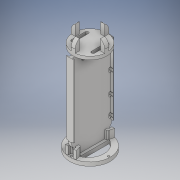
# Autodesk Inventor part: Platform_v1
Saved by Autodesk Inventor 2017 (Build 210142000, 142)
## iProperties
Created: 2018-06-09
Part Number: Platform_v1
Material: Generic
Document SubType Name: Modeling
Designer: Arthur
Density: 1 g/cm^3
Appearance: Default
Author: Arthur
Autodesk Inventor part; units mm, degrees
ref_plane "YZ Plane" through (0, 0, 0) normal (1, 0, 0) x (0, 1, 0)
ref_plane "XZ Plane" through (0, 0, 0) normal (0, 1, 0) x (-1, 0, 0)
ref_plane "XY Plane" through (0, 0, 0) normal (0, 0, 1) x (1, 0, 0)
sketch "Sketch3" plane through (0, 0, 0) normal (0, 1, 0) x (-1, 0, 0)
  circle A0 centre (0, 0) radius 37.75
  circle A1 centre (-34.675, 0) radius 1.9
  circle A2 centre (0, 34.675) radius 1.9
  circle A3 centre (34.675, 0) radius 1.9
  circle A4 centre (0, -34.675) radius 1.9
  line L0 (8, -27.7356) -> (8, 27.5985)
  arc A5 (8, -27.7356) -> (8, 27.5985) centre (-3.5989, -0.0685) ccw
  line L1 (-8, -27.7356) -> (-8, 27.5985)
  arc A6 (-8, 27.5985) -> (-8, -27.7356) centre (3.5989, -0.0685) ccw
  dimension "d3" = 3.8
  dimension "d7" = 3.8
  dimension "d9" = 3.8
  dimension "d33" = 30
  constraints: 7 centre point, 4 end point, 4 point on circle, 2 vertical
  measures "d3" diameter of A1
  measures "d7" diameter of A3
  measures "d9" diameter of A4
  measures "d33" radius of A6
extrude "Extrusion1" add sketch "Sketch3" along normal blind 7
sketch "Sketch4" plane through (0, 7, 0) normal (0, 1, 0) x (1, 0, 0)
  line L0 (-3, -30) -> (3, -30)
  line L1 (3, -24.5985) -> (3, 24.7356)
  line L2 (3, 30) -> (-3, 30)
  line L3 (-3, 24.7356) -> (-3, -24.2326)
  line L4 (-3, -30) -> (3, 30) construction
  line L5 (3, -30) -> (-3, 30) construction
  line L6 (-3, 30) -> (-5, 30)
  line L7 (-5, 30) -> (-5, 36)
  line L8 (-5, 36) -> (-10, 36)
  line L9 (-8, 27.7356) -> (-8, -27.5985) projected
  line L10 (-10, 36) -> (-8, 27.7356)
  line L11 (-3, -30) -> (-5, -30)
  line L12 (-5, -30) -> (-5, -36)
  line L13 (-5, -36) -> (-10, -36)
  line L14 (-10, -36) -> (-8, -27.2326)
  line L15 (-8, -27.2326) -> (-8, -24.2326)
  line L16 (-8, -24.2326) -> (-3, -24.2326)
  line L17 (-8, 27.7356) -> (-8, 24.7356)
  line L18 (-8, 24.7356) -> (-3, 24.7356)
  line L19 (3, -30) -> (5, -30)
  line L20 (5, -30) -> (5, -36)
  line L21 (5, -36) -> (10, -36)
  line L22 (10, -36) -> (8, -27.5985)
  line L23 (8, -27.5985) -> (8, -24.5985)
  line L24 (8, -27.5985) -> (8, 27.7356) projected
  line L25 (8, -24.5985) -> (5, -24.5985)
  line L26 (3, 30) -> (5, 30)
  line L27 (5, 30) -> (5, 36)
  line L28 (5, 36) -> (10, 36)
  line L29 (10, 36) -> (8, 27.7356)
  line L30 (8, 24.7356) -> (3, 24.7356)
  line L31 (5, -24.5985) -> (3, -24.5985)
  point P0 (0, 0)
  dimension "d36" = 6
  dimension "d37" = 60
  dimension "d38" = 2
  dimension "d39" = 6
  dimension "d40" = 5
  dimension "d41" = 6
  dimension "d42" = 5
  dimension "d43" = 3
  dimension "d44" = 3
  dimension "d45" = 2
  dimension "d46" = 5
  dimension "d47" = 3
  dimension "d48" = 2
  constraints: 60 end point, 13 perpendicular, 6 horizontal, 5 point on line, 2 midpoint, 2 parallel
  measures "d36" distance of L2.end L2.start
  measures "d37" distance of L2.start L0.end
  measures "d38" distance of L2.end L6.end
  measures "d39" distance of L6.end L7.end
  measures "d40" distance of L7.end L8.end
  measures "d41" distance of L11.end L12.end
  measures "d42" distance of L12.end L13.end
  measures "d43" distance of L14.end L15.end
  measures "d44" distance of L9.start L17.end
  measures "d45" distance of L0.end L19.end
  measures "d46" distance of L20.end L21.end
  measures "d47" distance of L22.end L23.end
  measures "d48" distance of L2.start L26.end
extrude "Extrusion2" add sketch "Sketch4" along normal blind 15 contours L11 L12 L13 L14 L9 L16 L3 L18 L10 L8 L7 L6 L2 L26 L27 L28 L29 L24 L30 L1 L31 L25 L23 L22 L21 L20 L19 L0
fillet "Fillet1" radius 2 1 edges at (-5, 14.5, 30)
fillet "Fillet2" radius 2 1 edges at (5, 14.5, 30)
fillet "Fillet3" radius 2 1 edges at (-5, 14.5, -30)
fillet "Fillet4" radius 2 1 edges at (5, 14.5, -30)
fillet "Fillet5" radius 2 1 edges at (-8, 14.5, -24.7356)
fillet "Fillet6" radius 2 1 edges at (8, 14.5, -24.7356)
fillet "Fillet7" radius 2 1 edges at (8, 14.5, 24.5985)
fillet "Fillet8" radius 2 1 edges at (-8, 14.5, 24.2326)
sketch "Sketch5" plane through (0, 22, 0) normal (0, 1, 0) x (1, 0, 0)
  circle A0 centre (0, 0) radius 37.75 projected
  line L0 (3, -37.6306) -> (3, 37.6306)
  line L1 (-3, 37.6306) -> (-3, -37.6306)
  arc A1 (-3, -37.6306) -> (3, -37.6306) centre (0, 0) ccw
  arc A2 (3, 37.6306) -> (-3, 37.6306) centre (0, 0) ccw
  constraints: 4 end point, 4 point on circle, 2 centre point, 1 coincident, 1 parallel, 2 other
extrude "Extrusion3" add sketch "Sketch5" along normal blind 146 contours L0 A0 L1
fillet "Fillet9" radius 7 1 edges at (0, 22, 30)
fillet "Fillet10" radius 7 1 edges at (0, 22, -30)
fillet "Fillet11" radius 15 1 edges at (0, 22, 37.75)
fillet "Fillet12" radius 15 1 edges at (0, 22, -37.75)
sketch "Sketch8" plane through (0, 168, 0) normal (0, 1, 0) x (1, 0, 0)
  circle A0 centre (0, 0) radius 31.6345
  constraints: 1 centre point, 1 coincident
extrude "Extrusion5" add sketch "Sketch8" along normal blind 6
sketch "Sketch10" plane through (0, 168, 0) normal (0, -1, 0) x (1, 0, 0)
  line L0 (-7, 37.0953) -> (-7, 36.1306)
  line L1 (-7, 36.1306) -> (-3, 36.1306)
  line L2 (-3, 36.1306) -> (-3, 37.6306)
  line L3 (7, 37.0953) -> (7, 36.1306)
  line L4 (7, 36.1306) -> (3, 36.1306)
  line L5 (3, 36.1306) -> (3, 37.6306)
  line L6 (7, -37.0953) -> (7, -36.1306)
  line L7 (7, -36.1306) -> (3, -36.1306)
  line L8 (3, -36.1306) -> (3, -37.6306)
  line L9 (-7, -37.0953) -> (-7, -36.1306)
  line L10 (-7, -36.1306) -> (-3, -36.1306)
  line L11 (-3, -36.1306) -> (-3, -37.6306)
  arc A0 (7, 37.0953) -> (3, 37.6306) centre (0, 0) ccw
  arc A1 (-3, 37.6306) -> (-7, 37.0953) centre (0, 0) ccw
  arc A2 (-7, -37.0953) -> (-3, -37.6306) centre (0, 0) ccw
  arc A3 (3, -37.6306) -> (7, -37.0953) centre (0, 0) ccw
  constraints: 24 end point, 8 point on circle, 4 centre point, 4 parallel, 1 coincident
extrude "Extrusion7" add sketch "Sketch10" along normal blind 135
sketch "Sketch11" plane through (-3, 7, -24.7356) normal (-1, 0, 0) x (0, 0, 1)
  line L0 (60.8662, 26) -> (61.8309, 26) projected
  line L1 (58.8662, 31) -> (58.8662, 36) construction
  line L2 (60.8662, 31) -> (60.8662, 36)
  line L3 (56.8662, 36) -> (56.8662, 31)
  arc A0 (56.8662, 31) -> (60.8662, 31) centre (58.8662, 31) ccw
  arc A1 (60.8662, 36) -> (56.8662, 36) centre (58.8662, 36) ccw
  line L4 (-9.5219, 31) -> (-9.5219, 36) construction
  line L5 (-7.5219, 31) -> (-7.5219, 36)
  line L6 (-11.5219, 36) -> (-11.5219, 31)
  arc A2 (-11.5219, 31) -> (-7.5219, 31) centre (-9.5219, 31) ccw
  arc A3 (-7.5219, 36) -> (-11.5219, 36) centre (-9.5219, 36) ccw
  line L7 (58.8662, 65.1959) -> (58.8662, 70.1959) construction
  line L8 (60.8662, 65.1959) -> (60.8662, 70.1959)
  line L9 (56.8662, 70.1959) -> (56.8662, 65.1959)
  arc A4 (56.8662, 65.1959) -> (60.8662, 65.1959) centre (58.8662, 65.1959) ccw
  arc A5 (60.8662, 70.1959) -> (56.8662, 70.1959) centre (58.8662, 70.1959) ccw
  line L10 (-9.5219, 65.1959) -> (-9.5219, 70.1959) construction
  line L11 (-7.5219, 65.1959) -> (-7.5219, 70.1959)
  line L12 (-11.5219, 70.1959) -> (-11.5219, 65.1959)
  arc A6 (-11.5219, 65.1959) -> (-7.5219, 65.1959) centre (-9.5219, 65.1959) ccw
  arc A7 (-7.5219, 70.1959) -> (-11.5219, 70.1959) centre (-9.5219, 70.1959) ccw
  line L13 (58.8662, 104.699) -> (58.8662, 109.699) construction
  line L14 (60.8662, 104.699) -> (60.8662, 109.699)
  line L15 (56.8662, 109.699) -> (56.8662, 104.699)
  arc A8 (56.8662, 104.699) -> (60.8662, 104.699) centre (58.8662, 104.699) ccw
  arc A9 (60.8662, 109.699) -> (56.8662, 109.699) centre (58.8662, 109.699) ccw
  line L16 (-9.5219, 104.699) -> (-9.5219, 109.699) construction
  line L17 (-7.5219, 104.699) -> (-7.5219, 109.699)
  line L18 (-11.5219, 109.699) -> (-11.5219, 104.699)
  arc A10 (-11.5219, 104.699) -> (-7.5219, 104.699) centre (-9.5219, 104.699) ccw
  arc A11 (-7.5219, 109.699) -> (-11.5219, 109.699) centre (-9.5219, 109.699) ccw
  line L19 (58.8662, 144.202) -> (58.8662, 149.202) construction
  line L20 (60.8662, 144.202) -> (60.8662, 149.202)
  line L21 (56.8662, 149.202) -> (56.8662, 144.202)
  arc A12 (56.8662, 144.202) -> (60.8662, 144.202) centre (58.8662, 144.202) ccw
  arc A13 (60.8662, 149.202) -> (56.8662, 149.202) centre (58.8662, 149.202) ccw
  line L22 (-9.5219, 144.202) -> (-9.5219, 149.202) construction
  line L23 (-7.5219, 144.202) -> (-7.5219, 149.202)
  line L24 (-11.5219, 149.202) -> (-11.5219, 144.202)
  arc A14 (-11.5219, 144.202) -> (-7.5219, 144.202) centre (-9.5219, 144.202) ccw
  arc A15 (-7.5219, 149.202) -> (-11.5219, 149.202) centre (-9.5219, 149.202) ccw
  point P0 (24.7356, -7)
  point P1 (58.8662, 33.5)
  point P2 (-9.5219, 33.5)
  point P3 (58.8662, 67.6959)
  point P4 (-9.5219, 67.6959)
  point P5 (58.8662, 107.199)
  point P6 (-9.5219, 107.199)
  point P7 (58.8662, 146.702)
  point P8 (-9.5219, 146.702)
  dimension "d90" = 5
  dimension "d91" = 4
  dimension "d94" = 4
  dimension "d95" = 5
  dimension "d96" = 4
  dimension "d97" = 4
  dimension "d98" = 5
  dimension "d99" = 4
  dimension "d100" = 4
  dimension "d101" = 5
  dimension "d102" = 4
  dimension "d103" = 4
  constraints: 64 end point, 32 point on circle, 32 tangent, 16 centre point, 8 midpoint, 8 parallel, 8 vertical
  measures "d90" distance of L1.start L1.end
  measures "d91" diameter of A1
  measures "d94" diameter of A3
  measures "d95" distance of L7.start L7.end
  measures "d96" diameter of A5
  measures "d97" diameter of A7
  measures "d98" distance of L13.start L13.end
  measures "d99" diameter of A9
  measures "d100" diameter of A11
  measures "d101" distance of L19.start L19.end
  measures "d102" diameter of A13
  measures "d103" diameter of A15
extrude "Extrusion8" cut sketch "Sketch11" against normal through all
sketch "Sketch13" plane through (0, 174, 0) normal (0, 1, 0) x (1, 0, 0)
  circle A0 centre (0, 0) radius 31.6345 projected
  line L0 (-23.6093, -3.9201) -> (-31.3907, -3.9201)
  line L1 (-31.3907, 3.9201) -> (-23.6093, 3.9201)
  line L2 (-23.6093, 3.9201) -> (-23.6093, -3.9201)
  line L3 (-3.6834, 23.5807) -> (3.6834, 23.5807)
  line L4 (3.6834, 23.5807) -> (3.6834, 31.4193)
  line L5 (-3.6834, 31.4193) -> (-3.6834, 23.5807)
  line L6 (-3.6834, -23.5807) -> (3.6834, -23.5807)
  line L7 (3.6834, -23.5807) -> (3.6834, -31.4193)
  line L8 (-3.6834, -31.4193) -> (-3.6834, -23.5807)
  line L9 (23.6093, -3.9201) -> (31.3907, -3.9201)
  line L10 (31.3907, 3.9201) -> (23.6093, 3.9201)
  line L11 (23.6093, 3.9201) -> (23.6093, -3.9201)
  arc A1 (-31.3907, 3.9201) -> (-31.3907, -3.9201) centre (0, 0) ccw
  arc A2 (-3.6834, -31.4193) -> (3.6834, -31.4193) centre (0, 0) ccw
  arc A3 (31.3907, -3.9201) -> (31.3907, 3.9201) centre (0, 0) ccw
  arc A4 (3.6834, 31.4193) -> (-3.6834, 31.4193) centre (0, 0) ccw
  point P0 (-27.5, 0)
  point P1 (0, 27.5)
  point P2 (0, -27.5)
  point P3 (27.5, 0)
  constraints: 24 end point, 8 point on circle, 4 centre point, 4 horizontal, 4 parallel, 2 perpendicular, 2 point on line, 2 other
extrude "Extrusion9" add sketch "Sketch13" along normal blind 20 contours A0 L9 L11 L10 | L4 L3 L5 A0 | A0 L8 L6 L7 | L1 L2 L0 A0
fillet "Fillet13" radius 15 4 edges at (-31.6345, 194, 0) (0, 194, -31.6345) (0, 194, 31.6345) (31.6345, 194, 0)
sketch "Sketch14" plane through (0, 174, 0) normal (0, 1, 0) x (1, 0, 0)
  line L0 (18.6342, -12.7219) -> (18.6342, 13) construction
  line L1 (21.6342, -12.7219) -> (21.6342, 13)
  line L2 (15.6342, 13) -> (15.6342, -12.7219)
  arc A0 (15.6342, -12.7219) -> (21.6342, -12.7219) centre (18.6342, -12.7219) ccw
  arc A1 (21.6342, 13) -> (15.6342, 13) centre (18.6342, 13) ccw
  line L3 (-18.8888, -13) -> (-18.8888, 13) construction
  line L4 (-15.8888, -13) -> (-15.8888, 13)
  line L5 (-21.8888, 13) -> (-21.8888, -13)
  arc A2 (-21.8888, -13) -> (-15.8888, -13) centre (-18.8888, -13) ccw
  arc A3 (-15.8888, 13) -> (-21.8888, 13) centre (-18.8888, 13) ccw
  point P0 (18.6342, 0.139)
  point P1 (-18.8888, 0)
  constraints: 16 end point, 8 point on circle, 8 tangent, 4 centre point, 2 midpoint, 2 parallel, 2 vertical
extrude "Extrusion10" cut sketch "Sketch14" against normal blind 6
sketch "Sketch15" plane through (-3, 7, -24.7356) normal (-1, 0, 0) x (0, 0, 1)
  line L0 (9.9934, 151.1866) -> (39.9934, 151.1866) construction
  line L1 (9.9934, 147.5282) -> (39.9934, 147.5282)
  line L2 (39.9934, 154.845) -> (9.9934, 154.845)
  arc A0 (9.9934, 154.845) -> (9.9934, 147.5282) centre (9.9934, 151.1866) ccw
  arc A1 (39.9934, 147.5282) -> (39.9934, 154.845) centre (39.9934, 151.1866) ccw
  point P0 (24.7356, -7)
  point P1 (24.9934, 151.1866)
  dimension "d118" = 30
  constraints: 8 end point, 4 point on circle, 4 tangent, 2 centre point, 1 horizontal, 1 midpoint, 1 parallel
  measures "d118" distance of L0.start L0.end
extrude "Extrusion11" cut sketch "Sketch15" against normal blind 6
body "Solid1"
